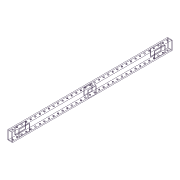
# Autodesk Inventor part: SideRail
Saved by Autodesk Inventor 2012 (Build 160160000, 160)
## iProperties
Created: 2012-10-20
Part Number: SideRail
Material: Aluminum-6061
Document SubType Name: Modeling
Designer: JesseK
Density: 2.71 g/cm^3
Mass: 1024.89 g
Surface Area: 2425.98 cm^2
Volume: 378.19 cm^3
Author: JesseK
Autodesk Inventor part; units mm, degrees
ref_plane "YZ Plane" through (0, 0, 0) normal (1, 0, 0) x (0, 1, 0)
ref_plane "XZ Plane" through (0, 0, 0) normal (0, 1, 0) x (-1, 0, 0)
ref_plane "XY Plane" through (0, 0, 0) normal (0, 0, 1) x (1, 0, 0)
sketch "Sketch1" plane through (0, 0, 0) normal (0, 0, 1) x (1, 0, 0)
  line L0 (0, 0) -> (-25.4, 0)
  line L1 (-25.4, 0) -> (-25.4, -50.8)
  line L2 (-25.4, -50.8) -> (0, -50.8)
  line L3 (0, -50.8) -> (0, 0)
  line L4 (-3.175, -3.175) -> (-22.225, -3.175)
  line L5 (-22.225, -3.175) -> (-22.225, -47.625)
  line L6 (-22.225, -47.625) -> (-3.175, -47.625)
  line L7 (-3.175, -47.625) -> (-3.175, -3.175)
  dimension "d0" = 25.4
  dimension "d1" = 50.8
  dimension "d2" = 3.175
  dimension "d3" = 3.175
  dimension "d4" = 3.175
  dimension "d5" = 3.175
  constraints: 16 end point, 4 parallel, 2 horizontal, 2 perpendicular
  measures "d0" distance of L0.start L0.end
  measures "d1" distance of L0.end L1.end
  measures "d2" distance between parallel lines of L3 L7
  measures "d3" distance between parallel lines of L0 L4
  measures "d4" distance between parallel lines of L1 L5
  measures "d5" distance between parallel lines of L2 L6
extrude "Extrusion1" add sketch "Sketch1" along normal blind 889
sketch "Sketch2" plane through (0, -50.8, 0) normal (1, 0, 0) x (0, 0, -1)
  line L0 (-889, 50.8) -> (-889, 0) projected
  line L1 (0, 0) -> (-889, 0) projected
  line L2 (-850.9, 44.45) -> (-793.75, 44.45)
  line L3 (-793.75, 44.45) -> (-793.75, 6.35)
  line L4 (-793.75, 6.35) -> (-850.9, 6.35)
  line L5 (-850.9, 6.35) -> (-850.9, 44.45)
  line L6 (-38.1, 44.45) -> (-95.25, 44.45)
  line L7 (-95.25, 44.45) -> (-95.25, 6.35)
  line L8 (-95.25, 6.35) -> (-38.1, 6.35)
  line L9 (-38.1, 6.35) -> (-38.1, 44.45)
  line L10 (0, 0) -> (0, 50.8) construction
  line L11 (-422.503, 41.275) -> (-466.497, 41.275)
  line L12 (-466.497, 41.275) -> (-466.497, 3.175)
  line L13 (-466.497, 3.175) -> (-422.503, 3.175)
  line L14 (-422.503, 3.175) -> (-422.503, 41.275)
  line L15 (-889, 41.275) -> (-466.497, 41.275) construction
  line L16 (-422.503, 47.625) -> (0, 47.625) construction
  line L17 (-433.5015, 41.275) -> (-422.503, 22.225) construction
  line L18 (-422.503, 22.225) -> (-433.5015, 3.175) construction
  line L19 (-433.5015, 3.175) -> (-455.4985, 3.175) construction
  line L20 (-455.4985, 3.175) -> (-466.497, 22.225) construction
  line L21 (-466.497, 22.225) -> (-455.4985, 41.275) construction
  line L22 (-455.4985, 41.275) -> (-433.5015, 41.275) construction
  line L23 (-422.503, 22.225) -> (0, 22.225) construction
  line L24 (-466.497, 22.225) -> (-889, 22.225) construction
  point P0 (-428.0022, 34.925)
  point P1 (-444.5, 41.275)
  point P2 (-444.5, 22.225)
  dimension "d8" = 38.1
  dimension "d9" = 57.15
  dimension "d10" = 6.35
  dimension "d11" = 38.1
  dimension "d14" = 38.1
  dimension "d15" = 57.15
  dimension "d16" = 38.1
  dimension "d17" = 6.35
  dimension "d27" = 38.1
  dimension "d28" = 3.175
  constraints: 44 end point, 8 horizontal, 6 parallel, 4 point on line, 3 equal length, 3 midpoint, 3 perpendicular, 13 other
  measures "d8" distance of L4.end L2.start
  measures "d9" distance of L3.end L4.end
  measures "d10" distance between parallel lines of L1 L4
  measures "d11" distance between parallel lines of L0 L5
  measures "d14" distance between parallel lines of L10 L9
  measures "d15" distance of L6.start L6.end
  measures "d16" distance of L6.end L7.end
  measures "d17" distance between parallel lines of L1 L8
  measures "d27" distance between parallel lines of L19 L22
  measures "d28" distance between parallel lines of L1 L13
extrude "Extrusion2" cut sketch "Sketch2" against normal through all
sketch "Sketch4" plane through (-25.4, 0, 0) normal (0, 1, 0) x (1, 0, 0)
  line L0 (25.4, 0) -> (25.4, -889) projected
  line L1 (25.4, 0) -> (0, 0) projected
  circle A0 centre (12.7, -12.7) radius 3.175
  dimension "d19" = 6.35
  dimension "d20" = 12.7
  dimension "d21" = 12.7
  constraints: 1 centre point
  measures "d19" diameter of A0
  measures "d20" distance from line of L0 A0.centre
  measures "d21" distance from line of L1 A0.centre
extrude "Extrusion3" cut sketch "Sketch4" against normal through all
pattern_linear "Rectangular Pattern1" count 35 spacing 25.4 along (0, 0, 1) of "Extrusion3"
body "Solid1"
